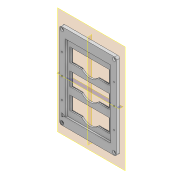
# Autodesk Inventor part: 30_xystage_gp-010b_adapter_slides
Saved by Autodesk Inventor 2022 (Build 260153000, 153)
## iProperties
Created: 2023-06-03
Part Number: 30_xystage_gp-010b_adapter_slides
Material: Generisch
Document SubType Name: Modeling
Designer: diederichbenedict
Density: 1 g/cm^3
Appearance: Vorgabe
Author: diederichbenedict
Autodesk Inventor part; units mm, degrees
ref_plane "YZ Plane" through (0, 0, 0) normal (1, 0, 0) x (0, 1, 0)
ref_plane "XZ Plane" through (0, 0, 0) normal (0, 1, 0) x (-1, 0, 0)
ref_plane "XY Plane" through (0, 0, 0) normal (0, 0, 1) x (1, 0, 0)
ref_plane "Arbeitsebene1" through (0, 0, 0) normal (0, 0, 1) x (1, 0, 0)
sketch "Skizze1" plane through (0, 0, 0) normal (0, 0, 1) x (1, 0, 0)
  line L0 (50, 77.5) -> (-50, 77.5) construction
  line L1 (-50, 77.5) -> (-50, -77.5) construction
  line L2 (-50, -77.5) -> (50, -77.5) construction
  line L3 (50, -77.5) -> (50, 77.5) construction
  line L4 (51, 82.5) -> (-51, 82.5)
  line L5 (-55, 78.5) -> (-55, -78.5)
  line L6 (-51, -82.5) -> (51, -82.5)
  line L7 (55, -78.5) -> (55, 78.5)
  circle A0 centre (50, 77.5) radius 1.6
  circle A1 centre (50, -77.5) radius 1.6
  circle A2 centre (-50, -77.5) radius 1.6
  circle A3 centre (-50, 77.5) radius 1.6
  arc A4 (55, 78.5) -> (51, 82.5) centre (51, 78.5) ccw
  arc A5 (51, -82.5) -> (55, -78.5) centre (51, -78.5) ccw
  arc A6 (-55, -78.5) -> (-51, -82.5) centre (-51, -78.5) ccw
  arc A7 (-51, 82.5) -> (-55, 78.5) centre (-51, 78.5) ccw
  line L8 (43, 64.5) -> (43, -64.5)
  line L9 (-43, -64.5) -> (-43, 64.5)
  line L10 (-43, 63.5) -> (-43, 64.5)
  line L11 (-43, 64.5) -> (43, 64.5)
  line L12 (43, 64.5) -> (43, 74.0537)
  line L13 (-43, -64.5) -> (43, -64.5)
  circle A8 centre (-43, 64.5) radius 5
  circle A9 centre (43, 64.5) radius 5
  circle A10 centre (43, -64.5) radius 5
  circle A11 centre (-43, -64.5) radius 5
  point P0 (0, 0)
  point P1 (-43, -59.5)
  point P2 (-43, 59.5)
  point P3 (-38, 64.5)
  point P4 (38, 64.5)
  point P5 (43, 59.5)
  point P6 (43, -59.5)
  point P7 (38, -64.5)
  point P8 (-38, -64.5)
  dimension "d1" = 3.2
  dimension "d2" = 3.2
  dimension "d3" = 3.2
  dimension "d4" = 3.2
  dimension "d5" = 4
  dimension "d6" = 86
  dimension "d10" = 10
  dimension "d11" = 10
  dimension "d12" = 10
  dimension "d13" = 10
  dimension "d31" = 43
  dimension "d32" = 129
  dimension "d33" = 100
  dimension "d34" = 155
  dimension "d35" = 64.5
  dimension "d36" = 55
  dimension "d37" = 110
  dimension "d38" = 165
  dimension "d39" = 82.5
  constraints: 28 end point, 12 centre point, 8 coincident, 8 point on circle, 8 tangent, 6 parallel, 3 equal radius, 2 perpendicular, 1 horizontal, 3 other
  measures "d1" diameter of A0
  measures "d2" diameter of A1
  measures "d3" diameter of A2
  measures "d4" diameter of A3
  measures "d5" radius of A4
  measures "d6" distance between parallel lines of L9 L8
  measures "d10" diameter of A8
  measures "d11" diameter of A9
  measures "d12" diameter of A10
  measures "d13" diameter of A11
  measures "d31" distance from line of point (0, 0) L8
  measures "d32" distance between parallel lines of L13 L11
  measures "d33" distance between parallel lines of L3 L1
  measures "d34" distance between parallel lines of L2 L0
  measures "d35" distance from line of point (0, 0) L11
  measures "d36" distance from line of L5 point (0, 0)
  measures "d37" distance between parallel lines of L7 L5
  measures "d38" distance between parallel lines of L6 L4
  measures "d39" distance from line of point (0, 0) L4
extrude "Extrusion1" add sketch "Skizze1" along normal blind 1 contours A4 L7 A5 L6 A6 L5 A7 L4 | L12 A9 L8 | L8 A9 L11 | L11 A9 L12 | L8 A10 L13 A11 L9 A8 L11 A9 | A10 L13 L8 | L8 L13 A10 | A8 L9 L11 | L11 L9 A8 | A11 L9 L13 | L13 L9 A11
sketch "Skizze2" plane through (0, 0, 1) normal (0, 0, 1) x (1, 0, 0)
  arc A0 (-51, 82.5) -> (-55, 78.5) centre (-51, 78.5) ccw projected
  line L0 (-55, 78.5) -> (-55, -78.5) projected
  arc A1 (-55, -78.5) -> (-51, -82.5) centre (-51, -78.5) ccw projected
  line L1 (-51, -82.5) -> (51, -82.5) projected
  arc A2 (51, -82.5) -> (55, -78.5) centre (51, -78.5) ccw projected
  line L2 (55, -78.5) -> (55, 78.5) projected
  arc A3 (55, 78.5) -> (51, 82.5) centre (51, 78.5) ccw projected
  line L3 (51, 82.5) -> (-51, 82.5) projected
  circle A4 centre (-50, 77.5) radius 1.6 projected
  circle A5 centre (-50, -77.5) radius 1.6 projected
  circle A6 centre (50, -77.5) radius 1.6 projected
  circle A7 centre (50, 77.5) radius 1.6 projected
  line L4 (-43, 64.5) -> (43, 64.5)
  line L5 (43, 64.5) -> (43, -64.5)
  line L6 (43, -64.5) -> (-43, -64.5)
  line L7 (-43, -64.5) -> (-43, 64.5)
  constraints: 8 end point, 2 parallel, 1 horizontal, 1 perpendicular
extrude "Extrusion2" add sketch "Skizze2" along normal blind 5 draft -5
sketch "Skizze3" plane through (0, 0, 6) normal (0, 0, 1) x (1, 0, 0)
  line L0 (-44.539, -64.7031) -> (-50.539, -68.1672)
  line L1 (-50.539, -68.1672) -> (-50.539, -61.239)
  line L2 (-50.539, -61.239) -> (-44.539, -64.7031)
  line L3 (39.5249, 74.6999) -> (39.5249, -55.3499) projected
  point P0 (0, 0)
  point P1 (-48.539, -64.7031)
  dimension "d23" = 6
  constraints: 6 end point, 7 other
  measures "d23" distance from line of L1 L0.start
extrude "Extrusion3" cut sketch "Skizze3" against normal blind 1
sketch "Skizze4" plane through (0, 0, 6) normal (0, 0, 1) x (1, 0, 0)
  line L0 (-44.539, -64.7031) -> (-50.539, -68.1672) projected
  line L1 (-50.539, -61.239) -> (-44.539, -64.7031) projected
  circle A0 centre (-50, 77.5) radius 2.0374 projected
  circle A1 centre (-50, -77.5) radius 2.0374 projected
  circle A2 centre (50, -77.5) radius 2.0374 projected
  circle A3 centre (50, 77.5) radius 2.0374 projected
  line L2 (-54.5626, -78.5) -> (-54.5626, 78.5) projected
  arc A4 (-54.5626, -78.5) -> (-51, -82.0626) centre (-51, -78.5) ccw projected
  line L3 (51, -82.0626) -> (-51, -82.0626) projected
  arc A5 (51, -82.0626) -> (54.5626, -78.5) centre (51, -78.5) ccw projected
  line L4 (54.5626, 78.5) -> (54.5626, -78.5) projected
  arc A6 (54.5626, 78.5) -> (51, 82.0626) centre (51, 78.5) ccw projected
  line L5 (-51, 82.0626) -> (51, 82.0626) projected
  arc A7 (-51, 82.0626) -> (-54.5626, 78.5) centre (-51, 78.5) ccw projected
  circle A8 centre (-50, -77.5) radius 1.6 projected
  circle A9 centre (50, -77.5) radius 1.6 projected
  circle A10 centre (50, 77.5) radius 1.6 projected
  circle A11 centre (-50, 77.5) radius 1.6 projected
  line L6 (-50.539, -68.1672) -> (-50.539, -61.239) projected
  point P0 (0, 0)
  constraints: 4 coincident
hole "Bohrung1" at (-50, -77.5, 6) at (50, -77.5, 6) at (50, 77.5, 6) at (-50, 77.5, 6) direction (0, 0, -1) diameter 3.2 end through all counterbore diameter 6.5 counterbore depth 3
sketch "Skizze7" plane through (0, 0, 6) normal (0, 0, 1) x (1, 0, 0)
  line L0 (-54.5626, -78.5) -> (-54.5626, 78.5) projected
  arc A0 (-54.5626, -78.5) -> (-51, -82.0626) centre (-51, -78.5) ccw projected
  line L1 (51, -82.0626) -> (-51, -82.0626) projected
  arc A1 (51, -82.0626) -> (54.5626, -78.5) centre (51, -78.5) ccw projected
  line L2 (54.5626, 78.5) -> (54.5626, -78.5) projected
  arc A2 (54.5626, 78.5) -> (51, 82.0626) centre (51, 78.5) ccw projected
  line L3 (-51, 82.0626) -> (51, 82.0626) projected
  arc A3 (-51, 82.0626) -> (-54.5626, 78.5) centre (-51, 78.5) ccw projected
  line L4 (-44.539, -64.7031) -> (-50.539, -68.1672) projected
  line L5 (-50.539, -68.1672) -> (-50.539, -61.239) projected
  line L6 (-50.539, -61.239) -> (-44.539, -64.7031) projected
  circle A4 centre (-50, 77.5) radius 3.25 projected
  circle A5 centre (50, -77.5) radius 3.25 projected
  circle A6 centre (-50, -77.5) radius 3.25 projected
  circle A7 centre (50, 77.5) radius 3.25 projected
  line L7 (-50, -81.5) -> (50, -81.5)
  line L8 (54, -77.5) -> (54, 77.5)
  line L9 (50, 81.5) -> (-50, 81.5)
  line L10 (-54, 77.5) -> (-54, -77.5)
  line L11 (-54, -81.5) -> (54, 81.5) construction
  line L12 (54, -81.5) -> (-54, 81.5) construction
  arc A8 (54, 77.5) -> (50, 81.5) centre (50, 77.5) ccw
  arc A9 (-50, 81.5) -> (-54, 77.5) centre (-50, 77.5) ccw
  arc A10 (-54, -77.5) -> (-50, -81.5) centre (-50, -77.5) ccw
  arc A11 (50, -81.5) -> (54, -77.5) centre (50, -77.5) ccw
  line L13 (43.4374, -64.9374) -> (-43.4374, -64.9374) projected
  line L14 (-43.4374, -64.9374) -> (-43.4374, 64.9374) projected
  line L15 (-43.4374, 64.9374) -> (43.4374, 64.9374) projected
  line L16 (43.4374, 64.9374) -> (43.4374, -64.9374) projected
  point P0 (0, 0)
  dimension "d52" = 108
  dimension "d53" = 163
  dimension "d54" = 4
  constraints: 12 end point, 8 point on circle, 8 point on line, 8 tangent, 4 centre point, 3 equal radius, 2 midpoint, 2 parallel, 1 horizontal, 1 perpendicular
  measures "d52" distance of L12.end L11.end
  measures "d53" distance of L11.end L12.start
  measures "d54" radius of A8
extrude "Extrusion6" cut sketch "Skizze7" against normal blind 10 contours L0 A3 L3 A2 L2 A1 L1 A0 | L4 L5 L6 | A4 | A5 | A6 | A7 | A10 L10 A9 L9 A8 L8 A11 L7 | L13 L14 L15 L16 keep common part
sketch "Skizze9" plane through (0, 0, 1) normal (0, 0, 1) x (1, 0, 0)
  line L0 (-35.5, -12.5) -> (35.5, -12.5)
  line L1 (35.5, -12.5) -> (35.5, 12.5)
  line L2 (35.5, 12.5) -> (-35.5, 12.5)
  line L3 (-35.5, 12.5) -> (-35.5, -12.5)
  line L4 (-35.5, -12.5) -> (35.5, 12.5) construction
  line L5 (35.5, -12.5) -> (-35.5, 12.5) construction
  arc A0 (-15.6125, -12.5) -> (15.6125, -12.5) centre (0, 0) ccw
  line L6 (-35.5, -52.5) -> (35.5, -52.5)
  line L7 (35.5, -52.5) -> (35.5, -27.5)
  line L8 (35.5, -27.5) -> (-35.5, -27.5)
  line L9 (-35.5, -27.5) -> (-35.5, -52.5)
  line L10 (-35.5, -52.5) -> (35.5, -27.5) construction
  line L11 (35.5, -52.5) -> (-35.5, -27.5) construction
  arc A1 (-15.6125, -52.5) -> (15.6125, -52.5) centre (0, -40) ccw
  line L12 (-35.5, 27.5) -> (35.5, 27.5)
  line L13 (35.5, 27.5) -> (35.5, 52.5)
  line L14 (35.5, 52.5) -> (-35.5, 52.5)
  line L15 (-35.5, 52.5) -> (-35.5, 27.5)
  line L16 (-35.5, 27.5) -> (35.5, 52.5) construction
  line L17 (35.5, 27.5) -> (-35.5, 52.5) construction
  arc A2 (-15.6125, 27.5) -> (15.6125, 27.5) centre (0, 40) ccw
  line L18 (-35.5, -12.5) -> (35.5, -12.5)
  line L19 (35.5, -12.5) -> (35.5, 12.5)
  line L20 (35.5, 12.5) -> (-35.5, 12.5)
  line L21 (-35.5, 12.5) -> (-35.5, -12.5)
  line L22 (-35.5, -12.5) -> (35.5, 12.5) construction
  line L23 (35.5, -12.5) -> (-35.5, 12.5) construction
  arc A3 (-15.6125, -12.5) -> (15.6125, -12.5) centre (0, 0) ccw
  dimension "d57" = 71
  dimension "d58" = 25
  dimension "d59" = 20
  dimension "d60" = 0
  dimension "d63" = 40
  dimension "d66" = 40
  constraints: 48 end point, 8 midpoint, 8 point on circle, 8 point on line, 4 centre point, 4 coincident, 2 collinear, 2 parallel, 2 vertical, 1 horizontal, 1 perpendicular, 46 other
  measures "d57" distance of L2.end L1.end
  measures "d58" distance of L1.end L0.end
  measures "d59" radius of A0
  measures "d60" distance of point (0, 0) point (0, 0)
  measures "d63" distance of point (0, 0) point (0, -40)
  measures "d66" distance of point (0, 0) point (0, 40)
extrude "Extrusion7" cut sketch "Skizze9" against normal blind 6
sketch "Skizze10" plane through (0, 0, 1) normal (0, 0, 1) x (1, 0, 0)
  circle A0 centre (50, 77.5) radius 3.25 projected
  circle A1 centre (-50, -77.5) radius 3.25 projected
  circle A2 centre (50, -77.5) radius 3.25 projected
  circle A3 centre (-50, 77.5) radius 3.25 projected
  line L0 (-44.539, -64.7031) -> (-50.539, -68.1672) projected
  line L1 (-50.539, -68.1672) -> (-50.539, -61.239) projected
  line L2 (-50.539, -61.239) -> (-44.539, -64.7031) projected
  line L3 (43.4374, 64.9374) -> (43.4374, -64.9374) projected
  line L4 (43.4374, -64.9374) -> (-43.4374, -64.9374) projected
  line L5 (-43.4374, -64.9374) -> (-43.4374, 64.9374) projected
  line L6 (-43.4374, 64.9374) -> (43.4374, 64.9374) projected
  line L7 (-54.5626, -78.5) -> (-54.5626, 78.5) projected
  arc A4 (-54.5626, -78.5) -> (-51, -82.0626) centre (-51, -78.5) ccw projected
  line L8 (51, -82.0626) -> (-51, -82.0626) projected
  arc A5 (51, -82.0626) -> (54.5626, -78.5) centre (51, -78.5) ccw projected
  line L9 (54.5626, 78.5) -> (54.5626, -78.5) projected
  arc A6 (54.5626, 78.5) -> (51, 82.0626) centre (51, 78.5) ccw projected
  line L10 (-51, 82.0626) -> (51, 82.0626) projected
  arc A7 (-51, 82.0626) -> (-54.5626, 78.5) centre (-51, 78.5) ccw projected
  arc A8 (-15.6125, -52.5) -> (15.6125, -52.5) centre (0, -40) ccw projected
  line L11 (-15.6125, -52.5) -> (-35.5, -52.5) projected
  line L12 (-35.5, -52.5) -> (-35.5, -27.5) projected
  line L13 (-35.5, -27.5) -> (35.5, -27.5) projected
  line L14 (35.5, -27.5) -> (35.5, -52.5) projected
  line L15 (35.5, -52.5) -> (15.6125, -52.5) projected
  arc A9 (-15.6125, -12.5) -> (15.6125, -12.5) centre (0, 0) ccw projected
  line L16 (-15.6125, -12.5) -> (-35.5, -12.5) projected
  line L17 (-35.5, -12.5) -> (-35.5, 12.5) projected
  line L18 (-35.5, 12.5) -> (35.5, 12.5) projected
  line L19 (35.5, 12.5) -> (35.5, -12.5) projected
  line L20 (35.5, -12.5) -> (15.6125, -12.5) projected
  arc A10 (-15.6125, 27.5) -> (15.6125, 27.5) centre (0, 40) ccw projected
  line L21 (-15.6125, 27.5) -> (-35.5, 27.5) projected
  line L22 (-35.5, 27.5) -> (-35.5, 52.5) projected
  line L23 (-35.5, 52.5) -> (35.5, 52.5) projected
  line L24 (35.5, 52.5) -> (35.5, 27.5) projected
  line L25 (35.5, 27.5) -> (15.6125, 27.5) projected
  line L26 (43, -64.5) -> (43, 64.5) projected
  line L27 (43, 64.5) -> (-43, 64.5) projected
  line L28 (-43, 64.5) -> (-43, -64.5) projected
  line L29 (-43, -64.5) -> (43, -64.5) projected
  line L30 (-38, 53) -> (38, 53)
  line L31 (38, 53) -> (38, 27)
  line L32 (38, 27) -> (-38, 27)
  line L33 (-38, 27) -> (-38, 53)
  line L34 (-38, 53) -> (38, 27) construction
  line L35 (38, 53) -> (-38, 27) construction
  line L36 (-38, -13) -> (-38, 13)
  line L37 (-38, 13) -> (38, 13)
  line L38 (-38, 13) -> (38, -13) construction
  line L39 (38, 13) -> (-38, -13) construction
  line L40 (38, -13) -> (-38, -13)
  line L41 (38, 13) -> (38, -13)
  line L42 (-38, -53) -> (-38, -27)
  line L43 (-38, -27) -> (38, -27)
  line L44 (-38, -27) -> (38, -53) construction
  line L45 (38, -27) -> (-38, -53) construction
  line L46 (38, -53) -> (-38, -53)
  line L47 (38, -27) -> (38, -53)
  point P0 (-35.5, 12.5)
  point P1 (-35.5, -12.5)
  point P2 (0, 0)
  point P3 (-15.6125, -12.5)
  point P4 (15.6125, -12.5)
  point P5 (35.5, 12.5)
  point P6 (35.5, -12.5)
  point P7 (0, -40)
  point P8 (15.1987, -53)
  point P9 (-15.1987, -53)
  point P10 (15.1987, -13)
  point P11 (-15.1987, -13)
  point P12 (15.1987, 27)
  point P13 (-15.1987, 27)
  dimension "d73" = 76
  dimension "d74" = 26
  dimension "d77" = 40
  constraints: 36 end point, 6 midpoint, 2 parallel, 1 collinear, 1 horizontal, 1 perpendicular, 1 vertical, 33 other
  measures "d73" distance of L31.end L32.end
  measures "d74" distance of L30.end L31.end
  measures "d77" distance of L30.start L36.end
extrude "Extrusion8" add sketch "Skizze10" along normal blind 2 contours L3 L4 L5 L6 | L29 L28 L27 L26
sketch "Skizze11" plane through (0, 0, 6) normal (0, 0, 1) x (1, 0, 0)
  line L0 (35.5, 12.5) -> (35.5, -12.5) projected
  line L1 (-35.5, -12.5) -> (-35.5, 12.5) projected
  circle A0 centre (50, 77.5) radius 3.25 projected
  circle A1 centre (-50, -77.5) radius 3.25 projected
  circle A2 centre (50, -77.5) radius 3.25 projected
  circle A3 centre (-50, 77.5) radius 3.25 projected
  line L2 (-44.539, -64.7031) -> (-50.539, -68.1672) projected
  line L3 (-50.539, -68.1672) -> (-50.539, -61.239) projected
  line L4 (-50.539, -61.239) -> (-44.539, -64.7031) projected
  line L5 (43.4374, 64.9374) -> (43.4374, -64.9374) projected
  line L6 (43.4374, -64.9374) -> (-43.4374, -64.9374) projected
  line L7 (-43.4374, -64.9374) -> (-43.4374, 64.9374) projected
  line L8 (-43.4374, 64.9374) -> (43.4374, 64.9374) projected
  line L9 (-54.5626, -78.5) -> (-54.5626, 78.5) projected
  arc A4 (-54.5626, -78.5) -> (-51, -82.0626) centre (-51, -78.5) ccw projected
  line L10 (51, -82.0626) -> (-51, -82.0626) projected
  arc A5 (51, -82.0626) -> (54.5626, -78.5) centre (51, -78.5) ccw projected
  line L11 (54.5626, 78.5) -> (54.5626, -78.5) projected
  arc A6 (54.5626, 78.5) -> (51, 82.0626) centre (51, 78.5) ccw projected
  line L12 (-51, 82.0626) -> (51, 82.0626) projected
  arc A7 (-51, 82.0626) -> (-54.5626, 78.5) centre (-51, 78.5) ccw projected
  circle A8 centre (50, 0) radius 1.4
  circle A9 centre (-50, 0) radius 1.4
  point P0 (0, 0)
  dimension "d84" = 2.8
  dimension "d85" = 2.8
  constraints: 2 centre point
  measures "d84" diameter of A8
  measures "d85" diameter of A9
extrude "Extrusion9" cut sketch "Skizze11" against normal through all contours A8 | A9
pattern_linear "Rechteckige Anordnung1" count 3 spacing 40 along (0, 1, 0) of "Extrusion9" first direction both ways yes
ref_plane "Arbeitsebene2" through (0, -78.5, 6) normal (1, 0, 0) x (0, 0, -1)
ref_plane "Arbeitsebene3" through (-51, 0, 6) normal (0, -1, 0) x (1, 0, 0)
equation "\"d11\" = d10"
equation "\"d12\" = d10"
equation "\"d13\" = d10"
equation "\"d31\" = 0.5 * d6"
equation "\"d35\" = 0.5 * d32"
equation "\"d36\" = 0.5 * d37"
equation "\"d39\" = 0.5 * d38"
